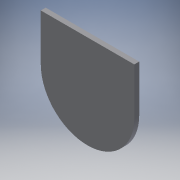
# Autodesk Inventor part: LargeConnectorBodies
Saved by Autodesk Inventor 2016 (Build 200138000, 138)
## iProperties
Created: 2017-03-11
Part Number: LargeConnectorBodies
Material: Generic
Document SubType Name: Modeling
Designer: Owner
Density: 1 g/cm^3
Appearance: Default
Author: Owner
Autodesk Inventor part; units mm, degrees
ref_plane "YZ Plane" through (0, 0, 0) normal (1, 0, 0) x (0, 1, 0)
ref_plane "XZ Plane" through (0, 0, 0) normal (0, 1, 0) x (-1, 0, 0)
ref_plane "XY Plane" through (0, 0, 0) normal (0, 0, 1) x (1, 0, 0)
sketch "Sketch1" plane through (0, 0, 0) normal (0, 0, 1) x (1, 0, 0)
  line L0 (-6.35, -214.55) -> (-6.35, -203.8154) projected
  line L1 (-6.35, -203.8154) -> (6.35, -203.8154) projected
  line L2 (6.35, -203.8154) -> (6.35, -214.55) projected
  line L3 (6.35, -214.55) -> (43.1, -214.55) projected
  line L4 (43.1, -214.55) -> (43.1, -189.15) projected
  line L5 (43.1, -189.15) -> (40.1028, -189.15) projected
  line L6 (40.1028, -189.15) -> (40.1028, -176.45) projected
  line L7 (40.1028, -176.45) -> (43.1, -176.45) projected
  line L8 (43.1, -176.45) -> (43.1, -110.25) projected
  line L9 (43.1, -110.25) -> (40.1028, -110.25) projected
  line L10 (40.1028, -110.25) -> (40.1028, -97.55) projected
  line L11 (40.1028, -97.55) -> (43.1, -97.55) projected
  line L12 (43.1, -97.55) -> (43.1, -72.15) projected
  line L13 (43.1, -72.15) -> (35.023, -72.15) projected
  arc A0 (-35.023, -72.15) -> (35.023, -72.15) centre (0, -57.15) ccw projected
  line L14 (-35.023, -72.15) -> (-43.1, -72.15) projected
  line L15 (-43.1, -72.15) -> (-43.1, -97.55) projected
  line L16 (-43.1, -97.55) -> (-40.1028, -97.55) projected
  line L17 (-40.1028, -97.55) -> (-40.1028, -110.25) projected
  line L18 (-40.1028, -110.25) -> (-43.1, -110.25) projected
  line L19 (-43.1, -110.25) -> (-43.1, -176.45) projected
  line L20 (-43.1, -176.45) -> (-40.1028, -176.45) projected
  line L21 (-40.1028, -176.45) -> (-40.1028, -189.15) projected
  line L22 (-40.1028, -189.15) -> (-43.1, -189.15) projected
  line L23 (-43.1, -189.15) -> (-43.1, -214.55) projected
  line L24 (-43.1, -214.55) -> (-6.35, -214.55) projected
  line L25 (-15.24, -146.85) -> (-11.16, -146.85) projected
  line L26 (-11.16, -146.85) -> (-11.16, -138.135) projected
  line L27 (-11.16, -138.135) -> (10.16, -138.135) projected
  line L28 (10.16, -138.135) -> (10.16, -168.265) projected
  line L29 (10.16, -168.265) -> (-11.16, -168.265) projected
  line L30 (-11.16, -168.265) -> (-11.16, -159.55) projected
  line L31 (-11.16, -159.55) -> (-19.058, -159.55) projected
  line L32 (-19.058, -159.55) -> (-19.058, -164.622) projected
  line L33 (-19.058, -164.622) -> (-22.598, -164.622) projected
  line L34 (-22.598, -164.622) -> (-22.598, -159.55) projected
  line L35 (-22.598, -159.55) -> (-32.258, -159.55) projected
  line L36 (-32.258, -159.55) -> (-32.258, -167.805) projected
  line L37 (-32.258, -167.805) -> (-34.29, -167.805) projected
  line L38 (-34.29, -167.805) -> (-34.29, -159.55) projected
  line L39 (-34.29, -159.55) -> (-38.1, -159.55) projected
  line L40 (-38.1, -159.55) -> (-38.1, -136.69) projected
  line L41 (-38.1, -136.69) -> (-22.598, -136.69) projected
  line L42 (-22.598, -136.69) -> (-22.598, -131.618) projected
  line L43 (-22.598, -131.618) -> (-19.058, -131.618) projected
  line L44 (-19.058, -131.618) -> (-19.058, -136.69) projected
  line L45 (-19.058, -136.69) -> (-15.24, -136.69) projected
  line L46 (-15.24, -136.69) -> (-15.24, -146.85) projected
  arc A1 (-38.1, -57.15) -> (38.1, -57.15) centre (0, -57.15) ccw projected
  line L47 (0, -57.15) -> (0, -82.55)
  circle A2 centre (0, -82.55) radius 38.1
  line L48 (38.1, -82.55) -> (-38.1, -82.55)
  line L49 (-38.1, -82.55) -> (-38.1, -44.45)
  line L50 (-38.1, -44.45) -> (38.1, -44.45)
  line L51 (38.1, -44.45) -> (38.1, -82.55)
  point P0 (0, 0)
  dimension "d1" = 76.2
  dimension "d0" = 25.4
  constraints: 10 end point, 2 parallel, 1 coincident, 1 horizontal, 1 horizontal alignment, 1 perpendicular, 1 vertical, 2 other
  measures "d0" distance of L47.start L47.end
extrude "Extrusion1" add sketch "Sketch1" along normal blind 4 contours L49 A1 A2 L14 | L14 A2 L49 | A2 A1 L14 | L14 A0 L48 A2 | L48 A0 A2 | L49 L50 A2 A1 | A1 A2 A0 L48 | L48 A0 L13 A2 | A2 L13 L51 | L48 A0 | L13 A2 A1 L51 | L50 L51 A1 A2 | L13 A1 A2
body "Solid1"
